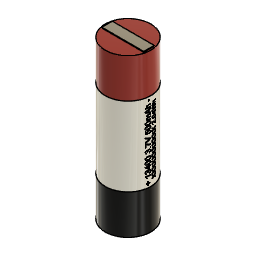
13400 lipo (Autodesk Fusion 360 design; units mm, degrees)
Autodesk Fusion 360 part; units mm, degrees
sketch "Sketch1" plane through (0, 0, 0) normal (0, 0, 1) x (1, 0, 0)
  circle A0 centre (0, 0) radius 6.5
  dimension "d1" = 13
  constraint coincident A0.centre origin
  measures "d1" diameter of A0
extrude "Extrude1" add sketch "Sketch1" along normal blind 11.25 makes body 1
extrude "Extrude2" add 1 faces at (1.9521, -0.9401, 11.25) along direction (0, 0, 1) blind 22.5 separate body on bodies 1 makes body 2
extrude "Extrude3" add 1 faces at (1.9521, -0.9401, 33.75) along direction (0, 0, 1) blind 11.25 separate body on bodies 2 makes body 3
sketch "Sketch2" plane through (0, 0, 45) normal (0, 0, 1) x (-1, 0, 0)
  circle A0 centre (0, 0) radius 6.5
  line L0 (6, 0) -> (6, 1.5)
  line L1 (6, 1.5) -> (6, -1.5)
  line L2 (6, 1.5) -> (-6, 1.5)
  line L3 (-6, 1.5) -> (-6, -1.5)
  line L4 (-6, -1.5) -> (6, -1.5)
  dimension "d8" = 6
  dimension "d9" = 3
  dimension "d10" = 12
  constraint perpendicular L1 L2
  constraint perpendicular L1 L4
  measures "d8" distance of A0.centre L0.start
  measures "d9" distance of L0.end L1.end
  measures "d10" distance of L0.end L2.end
extrude "Extrude4" add sketch "Sketch2" along normal blind 0.2 separate body contours L0 L1 L2 L3 L4 makes body 4
copy_body "CopyPasteBodies1" bodies 4 makes body 5
move_body "Move1" bodies 5 to x (1, 0, 0) y (0, 1, 0) z (0, 0, 1) at (0, 0, -45.2)
ref_plane "WorkPlane1" through (6.5, 0, 30.1907) normal (1, 0, 0) x (0, -1, 0)
sketch "Sketch3" plane through (6.5, 0, 30.1907) normal (1, 0, 0) x (0, 1, 0)
  line L0 (0, 2) -> (0, 3.56) construction
  line L1 (0, -18.94) -> (0, -17.38) construction
  line L2 (0, -17.38) -> (0, 2)
  line L3 (0, -17.38) -> (0.4, -17.38) construction
  line L4 (0.4, -17.38) -> (0.4, 2)
  dimension "d14" = 1.56
  dimension "d15" = 1.45
  dimension "d16" = 0.4
  dimension "d17" = 1.2
  text T0 "+ 13400 3.7V 500mAh -" font "Arial" height 1.45 align centre spacing 1 along the path L2 letters at x, y, angle (-1.8338, -18.4196, 90) (-1.8338, -17.2367, 90) (-1.8338, -16.6739, 90) (-1.8338, -15.5473, 90) (-1.8338, -14.4207, 90) (-1.8338, -13.2942, 90) (-1.8338, -12.1676, 90) (-1.8338, -11.041, 90) (-1.8338, -10.4782, 90) (-1.8338, -9.3517, 90) (-1.8338, -8.7889, 90) (-1.8338, -7.6623, 90) (-1.8338, -6.3112, 90) (-1.8338, -5.7484, 90) (-1.8338, -4.6219, 90) (-1.8338, -3.4953, 90) (-1.8338, -2.3687, 90) (-1.8338, -0.6813, 90) (-1.8338, 0.6757, 90) (-1.8338, 1.8023, 90) (-1.8338, 2.365, 90)
  text T1 "XXXXXXXXXXX 2.04Wh" font "Arial" height 1.2 align centre spacing 1 along the path L4 letters at x, y, angle (0.0824, -17.38, 90) (0.0824, -16.2126, 90) (0.0824, -15.0452, 90) (0.0824, -13.8778, 90) (0.0824, -12.7104, 90) (0.0824, -11.543, 90) (0.0824, -10.3756, 90) (0.0824, -9.2082, 90) (0.0824, -8.0408, 90) (0.0824, -6.8734, 90) (0.0824, -5.706, 90) (0.0824, -4.5386, 90) (0.0824, -4.0236, 90) (0.0824, -3.042, 90) (0.0824, -2.527, 90) (0.0824, -1.5454, 90) (0.0824, -0.5639, 90) (0.0824, 1.0677, 90)
  constraint vertical L0
  constraint vertical L1
  constraint parallel L0 L2
  constraint perpendicular L1 L3
  constraint perpendicular L3 L4
  measures "d14" distance of L1.start L1.end
  measures "d16" distance of L1.end L3.end
emboss "Emboss1" depth -0.01 profiles "Sketch3" section 1 text T1 T0 onto face at (6.4919, -0.324, 26.25) on bodies 2 bodies 2
move_body "Move2" bodies 1 3 2 4 5 to x (1, 0, 0) y (0, 1, 0) z (0, 0, 1) at (0, 0, 0.2)
equation "d2 = ( 45 / 4 ) * 1 mm"
equation "d4 = ( 45 / 4 ) * 2 mm"
equation "d6 = ( 45 / 4 ) * 1 mm"
equation "d9 = ( 1.500 * 2 ) * 1 mm"
named bodies: "Negative Wrap", "Center wrap", "Positive wrap", "Positive Terminal", "Negative Terminal"
